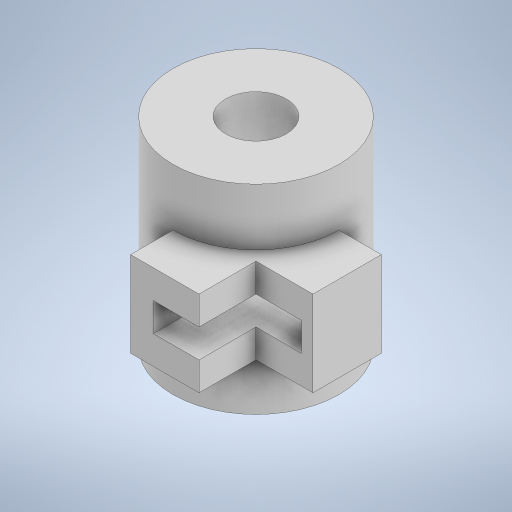
# Autodesk Inventor part: Sujetador
Saved by Autodesk Inventor 2024 (Build 280153000, 153)
## iProperties
Created: 2023-06-21
Part Number: Sujetador
Material: Genérico
Document SubType Name: Modeling
Designer: Personal
Density: 1 g/cm^3
Appearance: Valor por defecto
Author: Personal
Autodesk Inventor part; units mm, degrees
ref_plane "YZ Plane" through (0, 0, 0) normal (1, 0, 0) x (0, 1, 0)
ref_plane "XZ Plane" through (0, 0, 0) normal (0, 1, 0) x (-1, 0, 0)
ref_plane "XY Plane" through (0, 0, 0) normal (0, 0, 1) x (1, 0, 0)
sketch "Boceto1" plane through (0, 0, 0) normal (0, 1, 0) x (-1, 0, 0)
  circle A0 centre (0, 0) radius 5.3337
  circle A1 centre (0, 0) radius 14.5725
  constraints: 2 centre point, 2 coincident
extrude "Extrusión1" add sketch "Boceto1" along normal mid plane 35
sketch "Boceto2" plane through (0, 0, 0) normal (0, 1, 0) x (-1, 0, 0)
  line L0 (-12, 0) -> (-22, 0)
  line L1 (-22, 0) -> (-22, 12)
  line L2 (-22, 12) -> (-12, 12)
  line L3 (-12, 12) -> (-12, 22)
  line L4 (-12, 22) -> (0, 22)
  line L5 (0, 22) -> (0, 12)
  arc A0 (0, 12) -> (-12, 0) centre (0, 0) ccw
  line L6 (0, 0) -> (0, 23.3606) construction
  line L7 (0, 0) -> (-38.6088, 0) construction
  point P0 (0, 17)
  dimension "d4" = 10
  dimension "d5" = 12
  dimension "d6" = 10
  dimension "d7" = 12
  dimension "d10" = 10
  dimension "d11" = 10
  constraints: 16 end point, 4 perpendicular, 3 point on line, 2 horizontal, 2 point on circle, 2 vertical, 1 centre point, 1 collinear, 1 line through centre, 1 midpoint
  measures "d4" distance of L0.start L0.end
  measures "d5" distance of L0.end L1.end
  measures "d6" distance of L5.end L4.end
  measures "d7" distance of L3.end L4.end
  measures "d10" distance of L2.end L3.end
  measures "d11" distance of L1.end L2.end
extrude "Extrusión2" add sketch "Boceto2" along normal mid plane 15
sketch "Boceto3" plane through (0, 7.5, 22) normal (0, 0, 1) x (1, 0, 0)
  line L0 (4, -5) -> (12, -5)
  line L1 (12, -5) -> (12, -10)
  line L2 (12, -10) -> (4, -10)
  line L3 (4, -10) -> (4, -5)
  line L4 (12, -15) -> (12, 0) projected
  line L5 (12, -15) -> (0, -15) projected
  point P0 (0, -7.5)
  dimension "d8" = 5
  dimension "d9" = 5
  dimension "d14" = 8
  constraints: 8 end point, 2 parallel, 1 collinear, 1 horizontal, 1 perpendicular
  measures "d8" distance of L2.end L0.start
  measures "d9" distance between parallel lines of L5 L2
  measures "d14" distance of L0.start L0.end
extrude "Extrusión3" cut sketch "Boceto3" against normal blind 10
sketch "Boceto5" plane through (12, 7.5, 12) normal (0, 0, 1) x (1, 0, 0)
  point P0 (-12, -7.5)
sketch "Boceto6" plane through (12, 7.5, 12) normal (0, 0, 1) x (1, 0, 0)
  line L0 (-8, -10) -> (-8, -5) projected
  line L1 (-8, -5) -> (8, -5)
  line L2 (8, -5) -> (8, -10)
  line L3 (8, -10) -> (-8, -10)
  line L4 (-8, -10) -> (-8, -5)
  point P0 (-12, -7.5)
  point P1 (-8, -10)
  dimension "d19" = 16
  dimension "d20" = 5
  constraints: 8 end point, 2 parallel, 1 horizontal, 1 perpendicular
  measures "d19" distance of L0.end L1.end
  measures "d20" distance of L1.end L2.end
extrude "Extrusión5" cut sketch "Boceto6" against normal blind 10
